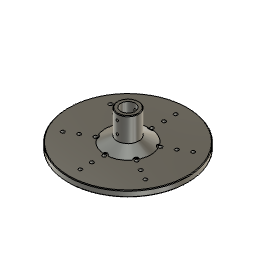
ピックアップチャッキ (Autodesk Fusion 360 design; units mm, degrees)
Autodesk Fusion 360 part; units mm, degrees
sketch "スケッチ1" plane through (0, 0, 0) normal (0, 0, 1) x (1, 0, 0)
  circle A0 centre (0, 0) radius 50
  dimension "d1" = 100
  constraint coincident A0.centre origin
  measures "d1" diameter of A0
extrude "押し出し1" add sketch "スケッチ1" along normal blind 5
sketch "スケッチ2" plane through (0, 0, 5) normal (0, 0, 1) x (-1, 0, 0)
  circle A0 centre (0, 0) radius 50
  circle A1 centre (0, 0) radius 9
  circle A2 centre (0, 0) radius 6
  dimension "d4" = 18
  dimension "d5" = 12
  constraint concentric A0 A1
  constraint coincident A0.centre A1.centre
  measures "d4" diameter of A1
  measures "d5" diameter of A2
extrude "押し出し2" add sketch "スケッチ2" along normal blind 25 contours A1
sketch "スケッチ3" plane through (0, 0, 0) normal (0, 1, 0) x (1, 0, 0)
  line L0 (9, -5) -> (9, -10)
  line L1 (9, -5) -> (19, -5)
  line L2 (19, -5) -> (9, -10)
  constraint vertical L0
  constraint perpendicular L0 L1
revolve "回転1" add sketch "スケッチ3" angle 360 about axis through (0, 0, 1.75) along (0, 0, 1)
chamfer "面取り1" distance 0.5 angle 45 3 edges at (-46.6164, -18.0808, 0) (-46.6164, -18.0808, 5) (8.3909, 3.2545, 30)
sketch "スケッチ4" plane through (0, 0, 0) normal (0, 1, 0) x (1, 0, 0)
  line L0 (0, -30) -> (0, -25)
  line L1 (0, -10) -> (0, -15)
  circle A0 centre (0, -25) radius 1
  circle A1 centre (0, -15) radius 1
  dimension "d10" = 2
  dimension "d11" = 2
  constraint vertical L0
  constraint vertical L1
  constraint coincident L0.end A0.centre
  constraint coincident L1.end A1.centre
  measures "d10" diameter of A0
  measures "d11" diameter of A1
extrude "押し出し3" cut sketch "スケッチ4" along normal blind 9 and the other way blind 9
sketch "スケッチ5" plane through (0, 0, 0) normal (0, 0, 1) x (1, 0, 0)
  circle A0 centre (0, -40) radius 1.5
  circle A1 centre (-0.2424, -30) radius 1.5
  circle A2 centre (0, -20) radius 1.5
  point P0 (0, -20)
  point P1 (0, -30)
  point P2 (0, -40)
  dimension "d16" = 3
  dimension "d17" = 3
  dimension "d18" = 3
  constraint coincident P2 A0.centre
  constraint coincident P0 A2.centre
  measures "d16" diameter of A0
  measures "d17" diameter of A1
  measures "d18" diameter of A2
extrude "押し出し4" cut sketch "スケッチ5" along normal blind 6
pattern_circular "C パターン1" count 6 over 360 about axis through (0, 0, 1.75) along (0, 0, 1) of 3 faces at (-1.4095, -39.487, 3.3333) (1.2502, -29.8506, 3.3333) (-1.1427, -19.0283, 3.3333)
sketch "スケッチ6" plane through (0, 0, 0) normal (0, 0, 1) x (1, 0, 0)
  circle A0 centre (0, 0) radius 1.5
  dimension "d23" = 3
  constraint coincident A0.centre origin
  measures "d23" diameter of A0
extrude "押し出し5" cut sketch "スケッチ6" along normal blind 5
sketch "スケッチ7" plane through (0, 0, 5) normal (0, 0, 1) x (-1, 0, 0)
  circle A0 centre (26.1019, 14.7901) radius 1.5
  circle A1 centre (25.8596, -15.2099) radius 1.5
  circle A2 centre (-0.2424, -30) radius 1.5
  circle A3 centre (-26.1019, -14.7901) radius 1.5
  circle A4 centre (-25.8596, 15.2099) radius 1.5
  circle A5 centre (34.641, 20) radius 1.5
  circle A6 centre (34.641, -20) radius 1.5
  circle A7 centre (0, -40) radius 1.5
  circle A8 centre (-34.641, -20) radius 1.5
  circle A9 centre (-34.641, 20) radius 1.5
  arc A10 (16.9721, 8.541) -> (15.8828, 10.4277) centre (17.3205, 10) ccw
  arc A11 (16.9721, -8.541) -> (16.9721, 8.541) centre (0, 0) ccw
  arc A12 (15.8828, -10.4277) -> (16.9721, -8.541) centre (17.3205, -10) ccw
  arc A13 (1.0893, -18.9688) -> (15.8828, -10.4277) centre (0, 0) ccw
  arc A14 (-1.0893, -18.9688) -> (1.0893, -18.9688) centre (0, -20) ccw
  arc A15 (-15.8828, -10.4277) -> (-1.0893, -18.9688) centre (0, 0) ccw
  arc A16 (-16.9721, -8.541) -> (-15.8828, -10.4277) centre (-17.3205, -10) ccw
  arc A17 (-16.9721, 8.541) -> (-16.9721, -8.541) centre (0, 0) ccw
  arc A18 (-15.8828, 10.4277) -> (-16.9721, 8.541) centre (-17.3205, 10) ccw
  arc A19 (-1.0893, 18.9688) -> (-15.8828, 10.4277) centre (0, 0) ccw
  arc A20 (1.0893, 18.9688) -> (-1.0893, 18.9688) centre (0, 20) ccw
  arc A21 (15.8828, 10.4277) -> (1.0893, 18.9688) centre (0, 0) ccw
  circle A22 centre (0.2424, 30) radius 1.5
  circle A23 centre (0, 40) radius 1.5
  circle A24 centre (0, 0) radius 49.5
  circle A25 centre (0, 20) radius 2.5
  circle A26 centre (-17.3205, 10) radius 2.5
  circle A27 centre (-17.3205, -10) radius 2.5
  circle A28 centre (0, -20) radius 2.5
  circle A29 centre (17.3205, -10) radius 2.5
  circle A30 centre (17.3205, 10) radius 2.5
  dimension "d26" = 5
  dimension "d28" = 360
  constraint concentric A20 A25
  measures "d26" diameter of A25
extrude "押し出し6" cut sketch "スケッチ7" along normal blind 1 contours A10 A11 A21 A30 | A11 A12 A13 A29 | A19 A20 A21 A25 | A13 A14 A15 A28 | A17 A18 A19 A26 | A15 A16 A17 A27 picked at (16.0359, 9.1878) picked at (16.0359, -9.1878) picked at (0.2115, 19.7656) picked at (-0.2115, -19.7656) picked at (-16.0331, 9.192) picked at (-17.2117, -9.7715)
